Autodesk Inventor part; units mm, degrees
(part 2 of 3)
  line L383 (87.0601, -26.6576) -> (86.7601, -26.6576)
  line L384 (84.5601, -24.0434) -> (84.5601, -7.2718)
  line L385 (89.5601, -7.2718) -> (89.5601, -24.0434)
  arc A154 (84.853, -6.5647) -> (84.5601, -7.2718) centre (85.5601, -7.2718) ccw
  line L386 (84.853, -6.5647) -> (86.7601, -4.6576)
  line L387 (87.0601, -4.6576) -> (86.7601, -4.6576)
  line L388 (87.0601, -4.6576) -> (87.3601, -4.6576)
  arc A155 (89.5601, -7.2718) -> (89.2672, -6.5647) centre (88.5601, -7.2718) ccw
  line L389 (89.2672, -6.5647) -> (87.3601, -4.6576)
  arc A156 (114.0672, 0.0495) -> (114.3601, 0.7566) centre (113.3601, 0.7566) ccw
  arc A157 (109.3601, 0.7566) -> (109.653, 0.0495) centre (110.3601, 0.7566) ccw
  line L390 (114.0672, 0.0495) -> (112.1601, -1.8576)
  line L391 (109.653, 0.0495) -> (111.5601, -1.8576)
  line L392 (111.8601, -1.8576) -> (112.1601, -1.8576)
  line L393 (111.8601, -1.8576) -> (111.5601, -1.8576)
  line L394 (109.3601, 0.7566) -> (109.3601, 17.5282)
  line L395 (114.3601, 17.5282) -> (114.3601, 0.7566)
  arc A158 (109.653, 18.2353) -> (109.3601, 17.5282) centre (110.3601, 17.5282) ccw
  line L396 (109.653, 18.2353) -> (111.5601, 20.1424)
  line L397 (111.8601, 20.1424) -> (111.5601, 20.1424)
  line L398 (111.8601, 20.1424) -> (112.1601, 20.1424)
  arc A159 (114.3601, 17.5282) -> (114.0672, 18.2353) centre (113.3601, 17.5282) ccw
  line L399 (114.0672, 18.2353) -> (112.1601, 20.1424)
  arc A160 (114.0672, -24.7505) -> (114.3601, -24.0434) centre (113.3601, -24.0434) ccw
  arc A161 (109.3601, -24.0434) -> (109.653, -24.7505) centre (110.3601, -24.0434) ccw
  line L400 (114.0672, -24.7505) -> (112.1601, -26.6576)
  line L401 (109.653, -24.7505) -> (111.5601, -26.6576)
  line L402 (111.8601, -26.6576) -> (112.1601, -26.6576)
  line L403 (111.8601, -26.6576) -> (111.5601, -26.6576)
  line L404 (109.3601, -24.0434) -> (109.3601, -7.2718)
  line L405 (114.3601, -7.2718) -> (114.3601, -24.0434)
  arc A162 (109.653, -6.5647) -> (109.3601, -7.2718) centre (110.3601, -7.2718) ccw
  line L406 (109.653, -6.5647) -> (111.5601, -4.6576)
  line L407 (111.8601, -4.6576) -> (111.5601, -4.6576)
  line L408 (111.8601, -4.6576) -> (112.1601, -4.6576)
  arc A163 (114.3601, -7.2718) -> (114.0672, -6.5647) centre (113.3601, -7.2718) ccw
  line L409 (114.0672, -6.5647) -> (112.1601, -4.6576)
  arc A164 (90.3672, -30.2647) -> (91.0743, -30.5576) centre (91.0743, -29.5576) ccw
  arc A165 (91.0743, -25.5576) -> (90.3672, -25.8505) centre (91.0743, -26.5576) ccw
  line L410 (90.3672, -30.2647) -> (88.4601, -28.3576)
  line L411 (90.3672, -25.8505) -> (88.4601, -27.7576)
  line L412 (88.4601, -28.0576) -> (88.4601, -28.3576)
  line L413 (88.4601, -28.0576) -> (88.4601, -27.7576)
  line L414 (91.0743, -25.5576) -> (107.8459, -25.5576)
  line L415 (107.8459, -30.5576) -> (91.0743, -30.5576)
  arc A166 (108.553, -25.8505) -> (107.8459, -25.5576) centre (107.8459, -26.5576) ccw
  line L416 (108.553, -25.8505) -> (110.4601, -27.7576)
  line L417 (110.4601, -28.0576) -> (110.4601, -27.7576)
  line L418 (110.4601, -28.0576) -> (110.4601, -28.3576)
  arc A167 (107.8459, -30.5576) -> (108.553, -30.2647) centre (107.8459, -29.5576) ccw
  line L419 (108.553, -30.2647) -> (110.4601, -28.3576)
  line L420 (-45.8399, 8.0424) -> (-44.8399, 8.0424)
  line L421 (-44.8399, 8.0424) -> (-42.8399, 6.0424)
  line L422 (-42.8399, 6.0424) -> (-42.8399, 5.0424)
  line L423 (-42.8399, 5.0424) -> (-44.8399, 3.0424)
  line L424 (-44.8399, 3.0424) -> (-45.8399, 3.0424)
  line L425 (-45.8399, 3.0424) -> (-47.8399, 5.0424)
  line L426 (-47.8399, 5.0424) -> (-47.8399, 6.0424)
  line L427 (-47.8399, 6.0424) -> (-45.8399, 8.0424)
  line L428 (-45.8399, -11.9576) -> (-44.8399, -11.9576)
  line L429 (-44.8399, -11.9576) -> (-42.8399, -13.9576)
  line L430 (-42.8399, -13.9576) -> (-42.8399, -14.9576)
  line L431 (-42.8399, -14.9576) -> (-44.8399, -16.9576)
  line L432 (-44.8399, -16.9576) -> (-45.8399, -16.9576)
  line L433 (-45.8399, -16.9576) -> (-47.8399, -14.9576)
  line L434 (-47.8399, -14.9576) -> (-47.8399, -13.9576)
  line L435 (-47.8399, -13.9576) -> (-45.8399, -11.9576)
  line L436 (38.2601, 8.0424) -> (39.2601, 8.0424)
  line L437 (39.2601, 8.0424) -> (41.2601, 6.0424)
  line L438 (41.2601, 6.0424) -> (41.2601, 5.0424)
  line L439 (41.2601, 5.0424) -> (39.2601, 3.0424)
  line L440 (39.2601, 3.0424) -> (38.2601, 3.0424)
  line L441 (38.2601, 3.0424) -> (36.2601, 5.0424)
  line L442 (36.2601, 5.0424) -> (36.2601, 6.0424)
  line L443 (36.2601, 6.0424) -> (38.2601, 8.0424)
  line L444 (38.2601, -11.9576) -> (39.2601, -11.9576)
  line L445 (39.2601, -11.9576) -> (41.2601, -13.9576)
  line L446 (41.2601, -13.9576) -> (41.2601, -14.9576)
  line L447 (41.2601, -14.9576) -> (39.2601, -16.9576)
  line L448 (39.2601, -16.9576) -> (38.2601, -16.9576)
  line L449 (38.2601, -16.9576) -> (36.2601, -14.9576)
  line L450 (36.2601, -14.9576) -> (36.2601, -13.9576)
  line L451 (36.2601, -13.9576) -> (38.2601, -11.9576)
  arc A168 (-143.5328, -5.6647) -> (-142.8257, -5.9576) centre (-142.8257, -4.9576) ccw
  arc A169 (-142.8257, -0.9576) -> (-143.5328, -1.2505) centre (-142.8257, -1.9576) ccw
  line L452 (-143.5328, -5.6647) -> (-145.4399, -3.7576)
  line L453 (-145.4399, -3.4576) -> (-145.4399, -3.1576)
  line L454 (-145.4399, -3.4576) -> (-145.4399, -3.7576)
  line L455 (-143.5328, -1.2505) -> (-145.4399, -3.1576)
  line L456 (-142.8257, -0.9576) -> (-132.0541, -0.9576)
  line L457 (-132.0541, -5.9576) -> (-142.8257, -5.9576)
  arc A170 (-131.347, -1.2505) -> (-132.0541, -0.9576) centre (-132.0541, -1.9576) ccw
  arc A171 (-132.0541, -5.9576) -> (-131.347, -5.6647) centre (-132.0541, -4.9576) ccw
  line L458 (-131.347, -5.6647) -> (-129.4399, -3.7576)
  line L459 (-129.4399, -3.4576) -> (-129.4399, -3.7576)
  line L460 (-129.4399, -3.4576) -> (-129.4399, -3.1576)
  line L461 (-131.347, -1.2505) -> (-129.4399, -3.1576)
  arc A172 (-144.2328, -0.5505) -> (-143.9399, 0.1566) centre (-144.9399, 0.1566) ccw
  arc A173 (-148.9399, 0.1566) -> (-148.647, -0.5505) centre (-147.9399, 0.1566) ccw
  line L462 (-144.2328, -0.5505) -> (-146.1399, -2.4576)
  line L463 (-146.4399, -2.4576) -> (-146.7399, -2.4576)
  line L464 (-146.4399, -2.4576) -> (-146.1399, -2.4576)
  line L465 (-148.647, -0.5505) -> (-146.7399, -2.4576)
  line L466 (-148.9399, 0.1566) -> (-148.9399, 10.9282)
  line L467 (-143.9399, 10.9282) -> (-143.9399, 0.1566)
  arc A174 (-148.647, 11.6353) -> (-148.9399, 10.9282) centre (-147.9399, 10.9282) ccw
  arc A175 (-143.9399, 10.9282) -> (-144.2328, 11.6353) centre (-144.9399, 10.9282) ccw
  line L468 (-144.2328, 11.6353) -> (-146.1399, 13.5424)
  line L469 (-146.4399, 13.5424) -> (-146.1399, 13.5424)
  line L470 (-146.4399, 13.5424) -> (-146.7399, 13.5424)
  line L471 (-148.647, 11.6353) -> (-146.7399, 13.5424)
  arc A176 (-161.5328, -5.6647) -> (-160.8257, -5.9576) centre (-160.8257, -4.9576) ccw
  arc A177 (-160.8257, -0.9576) -> (-161.5328, -1.2505) centre (-160.8257, -1.9576) ccw
  line L472 (-161.5328, -5.6647) -> (-163.4399, -3.7576)
  line L473 (-163.4399, -3.4576) -> (-163.4399, -3.1576)
  line L474 (-163.4399, -3.4576) -> (-163.4399, -3.7576)
  line L475 (-161.5328, -1.2505) -> (-163.4399, -3.1576)
  line L476 (-160.8257, -0.9576) -> (-150.0541, -0.9576)
  line L477 (-150.0541, -5.9576) -> (-160.8257, -5.9576)
  arc A178 (-149.347, -1.2505) -> (-150.0541, -0.9576) centre (-150.0541, -1.9576) ccw
  arc A179 (-150.0541, -5.9576) -> (-149.347, -5.6647) centre (-150.0541, -4.9576) ccw
  line L478 (-149.347, -5.6647) -> (-147.4399, -3.7576)
  line L479 (-147.4399, -3.4576) -> (-147.4399, -3.7576)
  line L480 (-147.4399, -3.4576) -> (-147.4399, -3.1576)
  line L481 (-149.347, -1.2505) -> (-147.4399, -3.1576)
  arc A180 (-144.2328, -18.5505) -> (-143.9399, -17.8434) centre (-144.9399, -17.8434) ccw
  arc A181 (-148.9399, -17.8434) -> (-148.647, -18.5505) centre (-147.9399, -17.8434) ccw
  line L482 (-144.2328, -18.5505) -> (-146.1399, -20.4576)
  line L483 (-146.4399, -20.4576) -> (-146.7399, -20.4576)
  line L484 (-146.4399, -20.4576) -> (-146.1399, -20.4576)
  line L485 (-148.647, -18.5505) -> (-146.7399, -20.4576)
  line L486 (-148.9399, -17.8434) -> (-148.9399, -7.0718)
  line L487 (-143.9399, -7.0718) -> (-143.9399, -17.8434)
  arc A182 (-148.647, -6.3647) -> (-148.9399, -7.0718) centre (-147.9399, -7.0718) ccw
  arc A183 (-143.9399, -7.0718) -> (-144.2328, -6.3647) centre (-144.9399, -7.0718) ccw
  line L488 (-144.2328, -6.3647) -> (-146.1399, -4.4576)
  line L489 (-146.4399, -4.4576) -> (-146.1399, -4.4576)
  line L490 (-146.4399, -4.4576) -> (-146.7399, -4.4576)
  line L491 (-148.647, -6.3647) -> (-146.7399, -4.4576)
  arc A184 (-170.0328, 10.3353) -> (-169.3257, 10.0424) centre (-169.3257, 11.0424) ccw
  arc A185 (-169.3257, 15.0424) -> (-170.0328, 14.7495) centre (-169.3257, 14.0424) ccw
  line L492 (-170.0328, 10.3353) -> (-171.9399, 12.2424)
  line L493 (-171.9399, 12.5424) -> (-171.9399, 12.8424)
  line L494 (-171.9399, 12.5424) -> (-171.9399, 12.2424)
  line L495 (-170.0328, 14.7495) -> (-171.9399, 12.8424)
  line L496 (-169.3257, 15.0424) -> (-158.5541, 15.0424)
  line L497 (-158.5541, 10.0424) -> (-169.3257, 10.0424)
  arc A186 (-157.847, 14.7495) -> (-158.5541, 15.0424) centre (-158.5541, 14.0424) ccw
  arc A187 (-158.5541, 10.0424) -> (-157.847, 10.3353) centre (-158.5541, 11.0424) ccw
  line L498 (-157.847, 10.3353) -> (-155.9399, 12.2424)
  line L499 (-155.9399, 12.5424) -> (-155.9399, 12.2424)
  line L500 (-155.9399, 12.5424) -> (-155.9399, 12.8424)
  line L501 (-157.847, 14.7495) -> (-155.9399, 12.8424)
  arc A188 (-187.0328, 10.3353) -> (-186.3257, 10.0424) centre (-186.3257, 11.0424) ccw
  arc A189 (-186.3257, 15.0424) -> (-187.0328, 14.7495) centre (-186.3257, 14.0424) ccw
  line L502 (-187.0328, 10.3353) -> (-188.9399, 12.2424)
  line L503 (-188.9399, 12.5424) -> (-188.9399, 12.8424)
  line L504 (-188.9399, 12.5424) -> (-188.9399, 12.2424)
  line L505 (-187.0328, 14.7495) -> (-188.9399, 12.8424)
  line L506 (-186.3257, 15.0424) -> (-175.5541, 15.0424)
  line L507 (-175.5541, 10.0424) -> (-186.3257, 10.0424)
  arc A190 (-174.847, 14.7495) -> (-175.5541, 15.0424) centre (-175.5541, 14.0424) ccw
  arc A191 (-175.5541, 10.0424) -> (-174.847, 10.3353) centre (-175.5541, 11.0424) ccw
  line L508 (-174.847, 10.3353) -> (-172.9399, 12.2424)
  line L509 (-172.9399, 12.5424) -> (-172.9399, 12.2424)
  line L510 (-172.9399, 12.5424) -> (-172.9399, 12.8424)
  line L511 (-174.847, 14.7495) -> (-172.9399, 12.8424)
  arc A192 (-170.2328, -3.0647) -> (-169.9399, -2.3576) centre (-170.9399, -2.3576) ccw
  arc A193 (-174.9399, -2.3576) -> (-174.647, -3.0647) centre (-173.9399, -2.3576) ccw
  line L512 (-170.2328, -3.0647) -> (-172.1399, -4.9718)
  line L513 (-172.4399, -4.9718) -> (-172.7399, -4.9718)
  line L514 (-172.4399, -4.9718) -> (-172.1399, -4.9718)
  line L515 (-174.647, -3.0647) -> (-172.7399, -4.9718)
  line L516 (-174.9399, -2.3576) -> (-174.9399, 8.414)
  line L517 (-169.9399, 8.414) -> (-169.9399, -2.3576)
  arc A194 (-174.647, 9.1211) -> (-174.9399, 8.414) centre (-173.9399, 8.414) ccw
  arc A195 (-169.9399, 8.414) -> (-170.2328, 9.1211) centre (-170.9399, 8.414) ccw
  line L518 (-170.2328, 9.1211) -> (-172.1399, 11.0282)
  line L519 (-172.4399, 11.0282) -> (-172.1399, 11.0282)
  line L520 (-172.4399, 11.0282) -> (-172.7399, 11.0282)
  line L521 (-174.647, 9.1211) -> (-172.7399, 11.0282)
  arc A196 (-170.2328, -19.5647) -> (-169.9399, -18.8576) centre (-170.9399, -18.8576) ccw
  arc A197 (-174.9399, -18.8576) -> (-174.647, -19.5647) centre (-173.9399, -18.8576) ccw
  line L522 (-170.2328, -19.5647) -> (-172.1399, -21.4718)
  line L523 (-172.4399, -21.4718) -> (-172.7399, -21.4718)
  line L524 (-172.4399, -21.4718) -> (-172.1399, -21.4718)
  line L525 (-174.647, -19.5647) -> (-172.7399, -21.4718)
  line L526 (-174.9399, -18.8576) -> (-174.9399, -8.086)
  line L527 (-169.9399, -8.086) -> (-169.9399, -18.8576)
  arc A198 (-174.647, -7.3789) -> (-174.9399, -8.086) centre (-173.9399, -8.086) ccw
  arc A199 (-169.9399, -8.086) -> (-170.2328, -7.3789) centre (-170.9399, -8.086) ccw
  line L528 (-170.2328, -7.3789) -> (-172.1399, -5.4718)
  line L529 (-172.4399, -5.4718) -> (-172.1399, -5.4718)
  line L530 (-172.4399, -5.4718) -> (-172.7399, -5.4718)
  line L531 (-174.647, -7.3789) -> (-172.7399, -5.4718)
  point P0 (-22.4267, -1.12)
  dimension "d362" = 7.5
  dimension "d363" = 17
  dimension "d364" = 7.5
  dimension "d365" = 17
  dimension "d366" = 7.5
  dimension "d367" = 0
  dimension "d368" = 0
  dimension "d369" = 0
  dimension "d370" = 0
  dimension "d371" = 0
  dimension "d372" = 15
  dimension "d373" = 0
  dimension "d374" = 16
  dimension "d375" = 6
  dimension "d376" = 6
  dimension "d377" = 13.6
  dimension "d378" = 16
  dimension "d379" = 6
  dimension "d380" = 15
  dimension "d381" = 0
  dimension "d509" = 23
  dimension "d510" = 25
  dimension "d511" = 24.6
  dimension "d514" = 0.5
sketch "Clock Front Face Outline" plane through (0, 0, 0) normal (0, 0, 1) x (1, 0, 0)
  line L0 (-365.1075, -11.3808) -> (-85.1075, -11.3808)
  line L1 (-60.1075, -36.3808) -> (-60.1075, -56.3808)
  line L2 (-85.1075, -81.3808) -> (-365.1075, -81.3808)
  line L3 (-390.1075, -56.3808) -> (-390.1075, -36.3808)
  arc A0 (-365.1075, -11.3808) -> (-390.1075, -36.3808) centre (-365.1075, -36.3808) ccw
  arc A1 (-60.1075, -36.3808) -> (-85.1075, -11.3808) centre (-85.1075, -36.3808) ccw
  arc A2 (-85.1075, -81.3808) -> (-60.1075, -56.3808) centre (-85.1075, -56.3808) ccw
  arc A3 (-390.1075, -56.3808) -> (-365.1075, -81.3808) centre (-365.1075, -56.3808) ccw
  point P0 (0, -2.2581)
  dimension "d429" = 330
  dimension "d430" = 70
  dimension "d431" = 25
  measures "d429" distance between parallel lines of L1 L3
  measures "d430" distance between parallel lines of L2 L0
  measures "d431" radius of A0
sketch "Small Segmemt" plane through (0, 0, 0) normal (0, 0, 1) x (1, 0, 0)
  arc A0 (-247.3536, -9.433) -> (-246.6465, -9.7259) centre (-246.6465, -8.7259) ccw
  arc A1 (-246.6465, -4.7259) -> (-247.3536, -5.0187) centre (-246.6465, -5.7259) ccw
  line L0 (-247.3536, -9.433) -> (-249.2607, -7.5259)
  line L1 (-249.2607, -7.2259) -> (-249.2607, -6.9259)
  line L2 (-249.2607, -7.2259) -> (-249.2607, -7.5259)
  line L3 (-247.3536, -5.0187) -> (-249.2607, -6.9259)
  line L4 (-246.6465, -4.7259) -> (-235.875, -4.7259)
  line L5 (-235.875, -9.7259) -> (-246.6465, -9.7259)
  arc A2 (-235.1679, -5.0187) -> (-235.875, -4.7259) centre (-235.875, -5.7259) ccw
  arc A3 (-235.875, -9.7259) -> (-235.1679, -9.433) centre (-235.875, -8.7259) ccw
  line L6 (-235.1679, -9.433) -> (-233.2607, -7.5259)
  line L7 (-233.2607, -7.2259) -> (-233.2607, -7.5259)
  line L8 (-233.2607, -7.2259) -> (-233.2607, -6.9259)
  line L9 (-235.1679, -5.0187) -> (-233.2607, -6.9259)
  point P0 (-225.4266, -6.7349)
  point P1 (-247.0607, -4.7259)
  point P2 (-247.0607, -9.7259)
  point P3 (-235.4607, -4.7259)
  point P4 (-235.4607, -9.7259)
  dimension "d462" = 2.2
  dimension "d463" = 2.2
  dimension "d464" = 2.2
  dimension "d465" = 2.2
  dimension "d466" = 2.2
  dimension "d467" = 2.2
  dimension "d468" = 2.2
  dimension "d469" = 1
  dimension "d470" = 5
  dimension "d471" = 2.2
  dimension "d472" = 2.2
  dimension "d473" = 135
  dimension "d474" = 16
  dimension "d475" = 135
  dimension "d476" = 2.5
  dimension "d477" = 5
  dimension "d478" = 16
  dimension "d479" = 2.2
  dimension "d480" = 0.3
  dimension "d481" = 0.3
  dimension "d482" = 0.3
  dimension "d483" = 0.3
  measures "d462" horizontal distance of point (-247.061, -9.726) L0.end
  measures "d463" horizontal distance of L8.end point (-235.461, -4.726)
  measures "d464" horizontal distance of point (-247.061, -4.726) L1.end
  measures "d465" horizontal distance of L6.end point (-235.461, -9.726)
  measures "d466" horizontal distance of L6.end point (-235.461, -9.726)
  measures "d467" horizontal distance of point (-247.061, -4.726) L1.end
  measures "d468" horizontal distance of point (-247.061, -9.726) L0.end
  measures "d469" radius of A1
  measures "d470" distance of point (-235.461, -9.726) point (-235.461, -4.726)
  measures "d471" horizontal distance of L8.end point (-235.461, -4.726)
  measures "d472" horizontal distance of point (-235.461, -9.726) L7.start
  measures "d473" angle of L5 L6
  measures "d474" horizontal distance of L6.end L1.start
  measures "d475" angle of L4 L9
  measures "d476" vertical distance of L7.start point (-235.461, -9.726)
  measures "d477" distance between parallel lines of L5 L4
  measures "d478" distance of L1.start L7.start
  measures "d479" horizontal distance of point (-247.061, -4.726) L1.start
  measures "d480" distance of L7.start L8.end
  measures "d481" distance of L6.end L7.start
  measures "d482" distance of L1.end L1.start
  measures "d483" distance of L0.end L1.start
sketch "Sketch1" plane through (0, 0, 0) normal (0, 0, 1) x (1, 0, 0)
  line L0 (-365.1075, -11.3808) -> (-85.1075, -11.3808)
  line L1 (-60.1075, -36.3808) -> (-60.1075, -56.3808)
  line L2 (-85.1075, -81.3808) -> (-365.1075, -81.3808)
  line L3 (-390.1075, -56.3808) -> (-390.1075, -36.3808)
  arc A0 (-365.1075, -11.3808) -> (-390.1075, -36.3808) centre (-365.1075, -36.3808) ccw
  arc A1 (-60.1075, -36.3808) -> (-85.1075, -11.3808) centre (-85.1075, -36.3808) ccw
  arc A2 (-85.1075, -81.3808) -> (-60.1075, -56.3808) centre (-85.1075, -56.3808) ccw
  arc A3 (-390.1075, -56.3808) -> (-365.1075, -81.3808) centre (-365.1075, -56.3808) ccw
  point P0 (0, 0)
extrude "Extrusion1" add sketch "Sketch1" along normal blind 3
sketch "Sketch5" plane through (0, 0, 3) normal (0, 0, 1) x (1, 0, 0)
  line L0 (-85.1075, -11.3808) -> (-365.1075, -11.3808) projected
  line L1 (-365.1075, -81.3808) -> (-85.1075, -81.3808) projected
  line L2 (-390.1075, -36.3808) -> (-390.1075, -56.3808) projected
  line L3 (-60.1075, -56.3808) -> (-60.1075, -36.3808) projected
  arc A0 (-136.1004, -24.0879) -> (-135.3933, -24.3808) centre (-135.3933, -23.3808) ccw
  arc A1 (-135.3933, -19.3808) -> (-136.1004, -19.6736) centre (-135.3933, -20.3808) ccw
  line L4 (-136.1004, -24.0879) -> (-138.0075, -22.1808)
  line L5 (-136.1004, -19.6736) -> (-138.0075, -21.5808)
  line L6 (-138.0075, -21.8808) -> (-138.0075, -22.1808)
  line L7 (-138.0075, -21.8808) -> (-138.0075, -21.5808)
  line L8 (-135.3933, -19.3808) -> (-118.6217, -19.3808)
  line L9 (-118.6217, -24.3808) -> (-135.3933, -24.3808)
  arc A2 (-117.9146, -19.6736) -> (-118.6217, -19.3808) centre (-118.6217, -20.3808) ccw
  line L10 (-117.9146, -19.6736) -> (-116.0075, -21.5808)
  line L11 (-116.0075, -21.8808) -> (-116.0075, -21.5808)
  line L12 (-116.0075, -21.8808) -> (-116.0075, -22.1808)
  arc A3 (-118.6217, -24.3808) -> (-117.9146, -24.0879) centre (-118.6217, -23.3808) ccw
  line L13 (-117.9146, -24.0879) -> (-116.0075, -22.1808)
  arc A4 (-136.1004, -48.8879) -> (-135.3933, -49.1808) centre (-135.3933, -48.1808) ccw
  arc A5 (-135.3933, -44.1808) -> (-136.1004, -44.4736) centre (-135.3933, -45.1808) ccw
  line L14 (-136.1004, -48.8879) -> (-138.0075, -46.9808)
  line L15 (-136.1004, -44.4736) -> (-138.0075, -46.3808)
  line L16 (-138.0075, -46.6808) -> (-138.0075, -46.9808)
  line L17 (-138.0075, -46.6808) -> (-138.0075, -46.3808)
  line L18 (-135.3933, -44.1808) -> (-118.6217, -44.1808)
  line L19 (-118.6217, -49.1808) -> (-135.3933, -49.1808)
  arc A6 (-117.9146, -44.4736) -> (-118.6217, -44.1808) centre (-118.6217, -45.1808) ccw
  line L20 (-117.9146, -44.4736) -> (-116.0075, -46.3808)
  line L21 (-116.0075, -46.6808) -> (-116.0075, -46.3808)
  line L22 (-116.0075, -46.6808) -> (-116.0075, -46.9808)
  arc A7 (-118.6217, -49.1808) -> (-117.9146, -48.8879) centre (-118.6217, -48.1808) ccw
  line L23 (-117.9146, -48.8879) -> (-116.0075, -46.9808)
  arc A8 (-137.2004, -43.3736) -> (-136.9075, -42.6665) centre (-137.9075, -42.6665) ccw
  arc A9 (-141.9075, -42.6665) -> (-141.6146, -43.3736) centre (-140.9075, -42.6665) ccw
  line L24 (-137.2004, -43.3736) -> (-139.1075, -45.2808)
  line L25 (-141.6146, -43.3736) -> (-139.7075, -45.2808)
  line L26 (-139.4075, -45.2808) -> (-139.1075, -45.2808)
  line L27 (-139.4075, -45.2808) -> (-139.7075, -45.2808)
  line L28 (-141.9075, -42.6665) -> (-141.9075, -25.895)
  line L29 (-136.9075, -25.895) -> (-136.9075, -42.6665)
  arc A10 (-141.6146, -25.1879) -> (-141.9075, -25.895) centre (-140.9075, -25.895) ccw
  line L30 (-141.6146, -25.1879) -> (-139.7075, -23.2808)
  line L31 (-139.4075, -23.2808) -> (-139.7075, -23.2808)
  line L32 (-139.4075, -23.2808) -> (-139.1075, -23.2808)
  arc A11 (-136.9075, -25.895) -> (-137.2004, -25.1879) centre (-137.9075, -25.895) ccw
  line L33 (-137.2004, -25.1879) -> (-139.1075, -23.2808)
  arc A12 (-137.2004, -68.1736) -> (-136.9075, -67.4665) centre (-137.9075, -67.4665) ccw
  arc A13 (-141.9075, -67.4665) -> (-141.6146, -68.1736) centre (-140.9075, -67.4665) ccw
  line L34 (-137.2004, -68.1736) -> (-139.1075, -70.0808)
  line L35 (-141.6146, -68.1736) -> (-139.7075, -70.0808)
  line L36 (-139.4075, -70.0808) -> (-139.1075, -70.0808)
  line L37 (-139.4075, -70.0808) -> (-139.7075, -70.0808)
  line L38 (-141.9075, -67.4665) -> (-141.9075, -50.695)
  line L39 (-136.9075, -50.695) -> (-136.9075, -67.4665)
  arc A14 (-141.6146, -49.9879) -> (-141.9075, -50.695) centre (-140.9075, -50.695) ccw
  line L40 (-141.6146, -49.9879) -> (-139.7075, -48.0808)
  line L41 (-139.4075, -48.0808) -> (-139.7075, -48.0808)
  line L42 (-139.4075, -48.0808) -> (-139.1075, -48.0808)
  arc A15 (-136.9075, -50.695) -> (-137.2004, -49.9879) centre (-137.9075, -50.695) ccw
  line L43 (-137.2004, -49.9879) -> (-139.1075, -48.0808)
  arc A16 (-112.4004, -43.3736) -> (-112.1075, -42.6665) centre (-113.1075, -42.6665) ccw
  arc A17 (-117.1075, -42.6665) -> (-116.8146, -43.3736) centre (-116.1075, -42.6665) ccw
  line L44 (-112.4004, -43.3736) -> (-114.3075, -45.2808)
  line L45 (-116.8146, -43.3736) -> (-114.9075, -45.2808)
  line L46 (-114.6075, -45.2808) -> (-114.3075, -45.2808)
  line L47 (-114.6075, -45.2808) -> (-114.9075, -45.2808)
  line L48 (-117.1075, -42.6665) -> (-117.1075, -25.895)
  line L49 (-112.1075, -25.895) -> (-112.1075, -42.6665)
  arc A18 (-116.8146, -25.1879) -> (-117.1075, -25.895) centre (-116.1075, -25.895) ccw
  line L50 (-116.8146, -25.1879) -> (-114.9075, -23.2808)
  line L51 (-114.6075, -23.2808) -> (-114.9075, -23.2808)
  line L52 (-114.6075, -23.2808) -> (-114.3075, -23.2808)
  arc A19 (-112.1075, -25.895) -> (-112.4004, -25.1879) centre (-113.1075, -25.895) ccw
  line L53 (-112.4004, -25.1879) -> (-114.3075, -23.2808)
  arc A20 (-112.4004, -68.1736) -> (-112.1075, -67.4665) centre (-113.1075, -67.4665) ccw
  arc A21 (-117.1075, -67.4665) -> (-116.8146, -68.1736) centre (-116.1075, -67.4665) ccw
  line L54 (-112.4004, -68.1736) -> (-114.3075, -70.0808)
  line L55 (-116.8146, -68.1736) -> (-114.9075, -70.0808)
  line L56 (-114.6075, -70.0808) -> (-114.3075, -70.0808)
  line L57 (-114.6075, -70.0808) -> (-114.9075, -70.0808)
  line L58 (-117.1075, -67.4665) -> (-117.1075, -50.695)
  line L59 (-112.1075, -50.695) -> (-112.1075, -67.4665)
  arc A22 (-116.8146, -49.9879) -> (-117.1075, -50.695) centre (-116.1075, -50.695) ccw
  line L60 (-116.8146, -49.9879) -> (-114.9075, -48.0808)
  line L61 (-114.6075, -48.0808) -> (-114.9075, -48.0808)
  line L62 (-114.6075, -48.0808) -> (-114.3075, -48.0808)
  arc A23 (-112.1075, -50.695) -> (-112.4004, -49.9879) centre (-113.1075, -50.695) ccw
  line L63 (-112.4004, -49.9879) -> (-114.3075, -48.0808)
  arc A24 (-136.1004, -73.6879) -> (-135.3933, -73.9808) centre (-135.3933, -72.9808) ccw
  arc A25 (-135.3933, -68.9808) -> (-136.1004, -69.2736) centre (-135.3933, -69.9808) ccw
  line L64 (-136.1004, -73.6879) -> (-138.0075, -71.7808)
  line L65 (-136.1004, -69.2736) -> (-138.0075, -71.1808)
  line L66 (-138.0075, -71.4808) -> (-138.0075, -71.7808)
  line L67 (-138.0075, -71.4808) -> (-138.0075, -71.1808)
  line L68 (-135.3933, -68.9808) -> (-118.6217, -68.9808)
  line L69 (-118.6217, -73.9808) -> (-135.3933, -73.9808)
  arc A26 (-117.9146, -69.2736) -> (-118.6217, -68.9808) centre (-118.6217, -69.9808) ccw
  line L70 (-117.9146, -69.2736) -> (-116.0075, -71.1808)
  line L71 (-116.0075, -71.4808) -> (-116.0075, -71.1808)
  line L72 (-116.0075, -71.4808) -> (-116.0075, -71.7808)
  arc A27 (-118.6217, -73.9808) -> (-117.9146, -73.6879) centre (-118.6217, -72.9808) ccw
  line L73 (-117.9146, -73.6879) -> (-116.0075, -71.7808)
  arc A28 (-182.9004, -24.0879) -> (-182.1933, -24.3808) centre (-182.1933, -23.3808) ccw
  arc A29 (-182.1933, -19.3808) -> (-182.9004, -19.6736) centre (-182.1933, -20.3808) ccw
  line L74 (-182.9004, -24.0879) -> (-184.8075, -22.1808)
  line L75 (-182.9004, -19.6736) -> (-184.8075, -21.5808)
  line L76 (-184.8075, -21.8808) -> (-184.8075, -22.1808)
  line L77 (-184.8075, -21.8808) -> (-184.8075, -21.5808)
  line L78 (-182.1933, -19.3808) -> (-165.4217, -19.3808)
  line L79 (-165.4217, -24.3808) -> (-182.1933, -24.3808)
  arc A30 (-164.7146, -19.6736) -> (-165.4217, -19.3808) centre (-165.4217, -20.3808) ccw
  line L80 (-164.7146, -19.6736) -> (-162.8075, -21.5808)
  line L81 (-162.8075, -21.8808) -> (-162.8075, -21.5808)
  line L82 (-162.8075, -21.8808) -> (-162.8075, -22.1808)
  arc A31 (-165.4217, -24.3808) -> (-164.7146, -24.0879) centre (-165.4217, -23.3808) ccw
  line L83 (-164.7146, -24.0879) -> (-162.8075, -22.1808)
  arc A32 (-182.9004, -48.8879) -> (-182.1933, -49.1808) centre (-182.1933, -48.1808) ccw
  arc A33 (-182.1933, -44.1808) -> (-182.9004, -44.4736) centre (-182.1933, -45.1808) ccw
  line L84 (-182.9004, -48.8879) -> (-184.8075, -46.9808)
  line L85 (-182.9004, -44.4736) -> (-184.8075, -46.3808)
  line L86 (-184.8075, -46.6808) -> (-184.8075, -46.9808)
  line L87 (-184.8075, -46.6808) -> (-184.8075, -46.3808)
  line L88 (-182.1933, -44.1808) -> (-165.4217, -44.1808)
  line L89 (-165.4217, -49.1808) -> (-182.1933, -49.1808)
  arc A34 (-164.7146, -44.4736) -> (-165.4217, -44.1808) centre (-165.4217, -45.1808) ccw
  line L90 (-164.7146, -44.4736) -> (-162.8075, -46.3808)
  line L91 (-162.8075, -46.6808) -> (-162.8075, -46.3808)
  line L92 (-162.8075, -46.6808) -> (-162.8075, -46.9808)
  arc A35 (-165.4217, -49.1808) -> (-164.7146, -48.8879) centre (-165.4217, -48.1808) ccw
  line L93 (-164.7146, -48.8879) -> (-162.8075, -46.9808)
  arc A36 (-184.0004, -43.3736) -> (-183.7075, -42.6665) centre (-184.7075, -42.6665) ccw
  arc A37 (-188.7075, -42.6665) -> (-188.4146, -43.3736) centre (-187.7075, -42.6665) ccw
  line L94 (-184.0004, -43.3736) -> (-185.9075, -45.2808)
  line L95 (-188.4146, -43.3736) -> (-186.5075, -45.2808)
  line L96 (-186.2075, -45.2808) -> (-185.9075, -45.2808)
  line L97 (-186.2075, -45.2808) -> (-186.5075, -45.2808)
  line L98 (-188.7075, -42.6665) -> (-188.7075, -25.895)
  line L99 (-183.7075, -25.895) -> (-183.7075, -42.6665)
  arc A38 (-188.4146, -25.1879) -> (-188.7075, -25.895) centre (-187.7075, -25.895) ccw
  line L100 (-188.4146, -25.1879) -> (-186.5075, -23.2808)
  line L101 (-186.2075, -23.2808) -> (-186.5075, -23.2808)
  line L102 (-186.2075, -23.2808) -> (-185.9075, -23.2808)
  arc A39 (-183.7075, -25.895) -> (-184.0004, -25.1879) centre (-184.7075, -25.895) ccw
  line L103 (-184.0004, -25.1879) -> (-185.9075, -23.2808)
  arc A40 (-184.0004, -68.1736) -> (-183.7075, -67.4665) centre (-184.7075, -67.4665) ccw
  arc A41 (-188.7075, -67.4665) -> (-188.4146, -68.1736) centre (-187.7075, -67.4665) ccw
  line L104 (-184.0004, -68.1736) -> (-185.9075, -70.0808)
  line L105 (-188.4146, -68.1736) -> (-186.5075, -70.0808)
  line L106 (-186.2075, -70.0808) -> (-185.9075, -70.0808)
  line L107 (-186.2075, -70.0808) -> (-186.5075, -70.0808)
  line L108 (-188.7075, -67.4665) -> (-188.7075, -50.695)
  line L109 (-183.7075, -50.695) -> (-183.7075, -67.4665)
  arc A42 (-188.4146, -49.9879) -> (-188.7075, -50.695) centre (-187.7075, -50.695) ccw
  line L110 (-188.4146, -49.9879) -> (-186.5075, -48.0808)
  line L111 (-186.2075, -48.0808) -> (-186.5075, -48.0808)
  line L112 (-186.2075, -48.0808) -> (-185.9075, -48.0808)
  arc A43 (-183.7075, -50.695) -> (-184.0004, -49.9879) centre (-184.7075, -50.695) ccw
  line L113 (-184.0004, -49.9879) -> (-185.9075, -48.0808)
  arc A44 (-159.2004, -43.3736) -> (-158.9075, -42.6665) centre (-159.9075, -42.6665) ccw
  arc A45 (-163.9075, -42.6665) -> (-163.6146, -43.3736) centre (-162.9075, -42.6665) ccw
  line L114 (-159.2004, -43.3736) -> (-161.1075, -45.2808)
  line L115 (-163.6146, -43.3736) -> (-161.7075, -45.2808)
  line L116 (-161.4075, -45.2808) -> (-161.1075, -45.2808)
  line L117 (-161.4075, -45.2808) -> (-161.7075, -45.2808)
  line L118 (-163.9075, -42.6665) -> (-163.9075, -25.895)
  line L119 (-158.9075, -25.895) -> (-158.9075, -42.6665)
  arc A46 (-163.6146, -25.1879) -> (-163.9075, -25.895) centre (-162.9075, -25.895) ccw
  line L120 (-163.6146, -25.1879) -> (-161.7075, -23.2808)
  line L121 (-161.4075, -23.2808) -> (-161.7075, -23.2808)
  line L122 (-161.4075, -23.2808) -> (-161.1075, -23.2808)
  arc A47 (-158.9075, -25.895) -> (-159.2004, -25.1879) centre (-159.9075, -25.895) ccw
  line L123 (-159.2004, -25.1879) -> (-161.1075, -23.2808)
  arc A48 (-159.2004, -68.1736) -> (-158.9075, -67.4665) centre (-159.9075, -67.4665) ccw
  arc A49 (-163.9075, -67.4665) -> (-163.6146, -68.1736) centre (-162.9075, -67.4665) ccw
  line L124 (-159.2004, -68.1736) -> (-161.1075, -70.0808)
  line L125 (-163.6146, -68.1736) -> (-161.7075, -70.0808)
  line L126 (-161.4075, -70.0808) -> (-161.1075, -70.0808)
  line L127 (-161.4075, -70.0808) -> (-161.7075, -70.0808)
  line L128 (-163.9075, -67.4665) -> (-163.9075, -50.695)
  line L129 (-158.9075, -50.695) -> (-158.9075, -67.4665)
  arc A50 (-163.6146, -49.9879) -> (-163.9075, -50.695) centre (-162.9075, -50.695) ccw
  line L130 (-163.6146, -49.9879) -> (-161.7075, -48.0808)
  line L131 (-161.4075, -48.0808) -> (-161.7075, -48.0808)
  line L132 (-161.4075, -48.0808) -> (-161.1075, -48.0808)
  arc A51 (-158.9075, -50.695) -> (-159.2004, -49.9879) centre (-159.9075, -50.695) ccw
  line L133 (-159.2004, -49.9879) -> (-161.1075, -48.0808)
  arc A52 (-182.9004, -73.6879) -> (-182.1933, -73.9808) centre (-182.1933, -72.9808) ccw
  arc A53 (-182.1933, -68.9808) -> (-182.9004, -69.2736) centre (-182.1933, -69.9808) ccw
  line L134 (-182.9004, -73.6879) -> (-184.8075, -71.7808)
  line L135 (-182.9004, -69.2736) -> (-184.8075, -71.1808)
  line L136 (-184.8075, -71.4808) -> (-184.8075, -71.7808)
  line L137 (-184.8075, -71.4808) -> (-184.8075, -71.1808)
  line L138 (-182.1933, -68.9808) -> (-165.4217, -68.9808)
  line L139 (-165.4217, -73.9808) -> (-182.1933, -73.9808)
  arc A54 (-164.7146, -69.2736) -> (-165.4217, -68.9808) centre (-165.4217, -69.9808) ccw
  line L140 (-164.7146, -69.2736) -> (-162.8075, -71.1808)
  line L141 (-162.8075, -71.4808) -> (-162.8075, -71.1808)
  line L142 (-162.8075, -71.4808) -> (-162.8075, -71.7808)
  arc A55 (-165.4217, -73.9808) -> (-164.7146, -73.6879) centre (-165.4217, -72.9808) ccw
  line L143 (-164.7146, -73.6879) -> (-162.8075, -71.7808)
  arc A56 (-220.2004, -24.0879) -> (-219.4933, -24.3808) centre (-219.4933, -23.3808) ccw
  arc A57 (-219.4933, -19.3808) -> (-220.2004, -19.6736) centre (-219.4933, -20.3808) ccw
  line L144 (-220.2004, -24.0879) -> (-222.1075, -22.1808)
  line L145 (-220.2004, -19.6736) -> (-222.1075, -21.5808)
  line L146 (-222.1075, -21.8808) -> (-222.1075, -22.1808)
  line L147 (-222.1075, -21.8808) -> (-222.1075, -21.5808)
  line L148 (-219.4933, -19.3808) -> (-202.7217, -19.3808)
  line L149 (-202.7217, -24.3808) -> (-219.4933, -24.3808)
  arc A58 (-202.0146, -19.6736) -> (-202.7217, -19.3808) centre (-202.7217, -20.3808) ccw
  line L150 (-202.0146, -19.6736) -> (-200.1075, -21.5808)
  line L151 (-200.1075, -21.8808) -> (-200.1075, -21.5808)
  line L152 (-200.1075, -21.8808) -> (-200.1075, -22.1808)
  arc A59 (-202.7217, -24.3808) -> (-202.0146, -24.0879) centre (-202.7217, -23.3808) ccw
  line L153 (-202.0146, -24.0879) -> (-200.1075, -22.1808)
  arc A60 (-220.2004, -48.8879) -> (-219.4933, -49.1808) centre (-219.4933, -48.1808) ccw
  arc A61 (-219.4933, -44.1808) -> (-220.2004, -44.4736) centre (-219.4933, -45.1808) ccw
  line L154 (-220.2004, -48.8879) -> (-222.1075, -46.9808)
  line L155 (-220.2004, -44.4736) -> (-222.1075, -46.3808)
  line L156 (-222.1075, -46.6808) -> (-222.1075, -46.9808)
  line L157 (-222.1075, -46.6808) -> (-222.1075, -46.3808)
  line L158 (-219.4933, -44.1808) -> (-202.7217, -44.1808)
  line L159 (-202.7217, -49.1808) -> (-219.4933, -49.1808)
  arc A62 (-202.0146, -44.4736) -> (-202.7217, -44.1808) centre (-202.7217, -45.1808) ccw
  line L160 (-202.0146, -44.4736) -> (-200.1075, -46.3808)
  line L161 (-200.1075, -46.6808) -> (-200.1075, -46.3808)
  line L162 (-200.1075, -46.6808) -> (-200.1075, -46.9808)
  arc A63 (-202.7217, -49.1808) -> (-202.0146, -48.8879) centre (-202.7217, -48.1808) ccw
  line L163 (-202.0146, -48.8879) -> (-200.1075, -46.9808)
  arc A64 (-221.3004, -43.3736) -> (-221.0075, -42.6665) centre (-222.0075, -42.6665) ccw
  arc A65 (-226.0075, -42.6665) -> (-225.7146, -43.3736) centre (-225.0075, -42.6665) ccw
  line L164 (-221.3004, -43.3736) -> (-223.2075, -45.2808)
  line L165 (-225.7146, -43.3736) -> (-223.8075, -45.2808)
  line L166 (-223.5075, -45.2808) -> (-223.2075, -45.2808)
  line L167 (-223.5075, -45.2808) -> (-223.8075, -45.2808)
  line L168 (-226.0075, -42.6665) -> (-226.0075, -25.895)
  line L169 (-221.0075, -25.895) -> (-221.0075, -42.6665)
  arc A66 (-225.7146, -25.1879) -> (-226.0075, -25.895) centre (-225.0075, -25.895) ccw
  line L170 (-225.7146, -25.1879) -> (-223.8075, -23.2808)
  line L171 (-223.5075, -23.2808) -> (-223.8075, -23.2808)
  line L172 (-223.5075, -23.2808) -> (-223.2075, -23.2808)
  arc A67 (-221.0075, -25.895) -> (-221.3004, -25.1879) centre (-222.0075, -25.895) ccw
  line L173 (-221.3004, -25.1879) -> (-223.2075, -23.2808)
  arc A68 (-221.3004, -68.1736) -> (-221.0075, -67.4665) centre (-222.0075, -67.4665) ccw
  arc A69 (-226.0075, -67.4665) -> (-225.7146, -68.1736) centre (-225.0075, -67.4665) ccw
  line L174 (-221.3004, -68.1736) -> (-223.2075, -70.0808)
  line L175 (-225.7146, -68.1736) -> (-223.8075, -70.0808)
  line L176 (-223.5075, -70.0808) -> (-223.2075, -70.0808)
  line L177 (-223.5075, -70.0808) -> (-223.8075, -70.0808)
  line L178 (-226.0075, -67.4665) -> (-226.0075, -50.695)
  line L179 (-221.0075, -50.695) -> (-221.0075, -67.4665)
  arc A70 (-225.7146, -49.9879) -> (-226.0075, -50.695) centre (-225.0075, -50.695) ccw
  line L180 (-225.7146, -49.9879) -> (-223.8075, -48.0808)
  line L181 (-223.5075, -48.0808) -> (-223.8075, -48.0808)
  line L182 (-223.5075, -48.0808) -> (-223.2075, -48.0808)
  arc A71 (-221.0075, -50.695) -> (-221.3004, -49.9879) centre (-222.0075, -50.695) ccw
  line L183 (-221.3004, -49.9879) -> (-223.2075, -48.0808)
  arc A72 (-196.5004, -43.3736) -> (-196.2075, -42.6665) centre (-197.2075, -42.6665) ccw
  arc A73 (-201.2075, -42.6665) -> (-200.9146, -43.3736) centre (-200.2075, -42.6665) ccw
  line L184 (-196.5004, -43.3736) -> (-198.4075, -45.2808)
  line L185 (-200.9146, -43.3736) -> (-199.0075, -45.2808)
  line L186 (-198.7075, -45.2808) -> (-198.4075, -45.2808)
  line L187 (-198.7075, -45.2808) -> (-199.0075, -45.2808)
  line L188 (-201.2075, -42.6665) -> (-201.2075, -25.895)
  line L189 (-196.2075, -25.895) -> (-196.2075, -42.6665)
  arc A74 (-200.9146, -25.1879) -> (-201.2075, -25.895) centre (-200.2075, -25.895) ccw
  line L190 (-200.9146, -25.1879) -> (-199.0075, -23.2808)
  line L191 (-198.7075, -23.2808) -> (-199.0075, -23.2808)
  line L192 (-198.7075, -23.2808) -> (-198.4075, -23.2808)
  arc A75 (-196.2075, -25.895) -> (-196.5004, -25.1879) centre (-197.2075, -25.895) ccw
  line L193 (-196.5004, -25.1879) -> (-198.4075, -23.2808)
  arc A76 (-196.5004, -68.1736) -> (-196.2075, -67.4665) centre (-197.2075, -67.4665) ccw
  arc A77 (-201.2075, -67.4665) -> (-200.9146, -68.1736) centre (-200.2075, -67.4665) ccw
  line L194 (-196.5004, -68.1736) -> (-198.4075, -70.0808)
  line L195 (-200.9146, -68.1736) -> (-199.0075, -70.0808)
  line L196 (-198.7075, -70.0808) -> (-198.4075, -70.0808)
  line L197 (-198.7075, -70.0808) -> (-199.0075, -70.0808)
  line L198 (-201.2075, -67.4665) -> (-201.2075, -50.695)
  line L199 (-196.2075, -50.695) -> (-196.2075, -67.4665)
  arc A78 (-200.9146, -49.9879) -> (-201.2075, -50.695) centre (-200.2075, -50.695) ccw
  line L200 (-200.9146, -49.9879) -> (-199.0075, -48.0808)
  line L201 (-198.7075, -48.0808) -> (-199.0075, -48.0808)
  line L202 (-198.7075, -48.0808) -> (-198.4075, -48.0808)
  arc A79 (-196.2075, -50.695) -> (-196.5004, -49.9879) centre (-197.2075, -50.695) ccw
  line L203 (-196.5004, -49.9879) -> (-198.4075, -48.0808)
  arc A80 (-220.2004, -73.6879) -> (-219.4933, -73.9808) centre (-219.4933, -72.9808) ccw
  arc A81 (-219.4933, -68.9808) -> (-220.2004, -69.2736) centre (-219.4933, -69.9808) ccw
  line L204 (-220.2004, -73.6879) -> (-222.1075, -71.7808)
  line L205 (-220.2004, -69.2736) -> (-222.1075, -71.1808)
  line L206 (-222.1075, -71.4808) -> (-222.1075, -71.7808)
  line L207 (-222.1075, -71.4808) -> (-222.1075, -71.1808)
  line L208 (-219.4933, -68.9808) -> (-202.7217, -68.9808)
  line L209 (-202.7217, -73.9808) -> (-219.4933, -73.9808)
  arc A82 (-202.0146, -69.2736) -> (-202.7217, -68.9808) centre (-202.7217, -69.9808) ccw
  line L210 (-202.0146, -69.2736) -> (-200.1075, -71.1808)
  line L211 (-200.1075, -71.4808) -> (-200.1075, -71.1808)
  line L212 (-200.1075, -71.4808) -> (-200.1075, -71.7808)
  arc A83 (-202.7217, -73.9808) -> (-202.0146, -73.6879) centre (-202.7217, -72.9808) ccw
  line L213 (-202.0146, -73.6879) -> (-200.1075, -71.7808)
  arc A84 (-267.0004, -24.0879) -> (-266.2933, -24.3808) centre (-266.2933, -23.3808) ccw
  arc A85 (-266.2933, -19.3808) -> (-267.0004, -19.6736) centre (-266.2933, -20.3808) ccw
  line L214 (-267.0004, -24.0879) -> (-268.9075, -22.1808)
  line L215 (-267.0004, -19.6736) -> (-268.9075, -21.5808)
  line L216 (-268.9075, -21.8808) -> (-268.9075, -22.1808)
  line L217 (-268.9075, -21.8808) -> (-268.9075, -21.5808)
  line L218 (-266.2933, -19.3808) -> (-249.5217, -19.3808)
  line L219 (-249.5217, -24.3808) -> (-266.2933, -24.3808)
  arc A86 (-248.8146, -19.6736) -> (-249.5217, -19.3808) centre (-249.5217, -20.3808) ccw
  line L220 (-248.8146, -19.6736) -> (-246.9075, -21.5808)
  line L221 (-246.9075, -21.8808) -> (-246.9075, -21.5808)
  line L222 (-246.9075, -21.8808) -> (-246.9075, -22.1808)
  arc A87 (-249.5217, -24.3808) -> (-248.8146, -24.0879) centre (-249.5217, -23.3808) ccw
  line L223 (-248.8146, -24.0879) -> (-246.9075, -22.1808)
  arc A88 (-267.0004, -48.8879) -> (-266.2933, -49.1808) centre (-266.2933, -48.1808) ccw
  arc A89 (-266.2933, -44.1808) -> (-267.0004, -44.4736) centre (-266.2933, -45.1808) ccw
  line L224 (-267.0004, -48.8879) -> (-268.9075, -46.9808)
  line L225 (-267.0004, -44.4736) -> (-268.9075, -46.3808)
  line L226 (-268.9075, -46.6808) -> (-268.9075, -46.9808)
  line L227 (-268.9075, -46.6808) -> (-268.9075, -46.3808)
  line L228 (-266.2933, -44.1808) -> (-249.5217, -44.1808)
  line L229 (-249.5217, -49.1808) -> (-266.2933, -49.1808)
  arc A90 (-248.8146, -44.4736) -> (-249.5217, -44.1808) centre (-249.5217, -45.1808) ccw
  line L230 (-248.8146, -44.4736) -> (-246.9075, -46.3808)
  line L231 (-246.9075, -46.6808) -> (-246.9075, -46.3808)
  line L232 (-246.9075, -46.6808) -> (-246.9075, -46.9808)
  arc A91 (-249.5217, -49.1808) -> (-248.8146, -48.8879) centre (-249.5217, -48.1808) ccw
  line L233 (-248.8146, -48.8879) -> (-246.9075, -46.9808)
  arc A92 (-268.1004, -43.3736) -> (-267.8075, -42.6665) centre (-268.8075, -42.6665) ccw
  arc A93 (-272.8075, -42.6665) -> (-272.5146, -43.3736) centre (-271.8075, -42.6665) ccw
  line L234 (-268.1004, -43.3736) -> (-270.0075, -45.2808)
  line L235 (-272.5146, -43.3736) -> (-270.6075, -45.2808)
  line L236 (-270.3075, -45.2808) -> (-270.0075, -45.2808)
  line L237 (-270.3075, -45.2808) -> (-270.6075, -45.2808)
  line L238 (-272.8075, -42.6665) -> (-272.8075, -25.895)
  line L239 (-267.8075, -25.895) -> (-267.8075, -42.6665)
  arc A94 (-272.5146, -25.1879) -> (-272.8075, -25.895) centre (-271.8075, -25.895) ccw
  line L240 (-272.5146, -25.1879) -> (-270.6075, -23.2808)
  line L241 (-270.3075, -23.2808) -> (-270.6075, -23.2808)
  line L242 (-270.3075, -23.2808) -> (-270.0075, -23.2808)
  arc A95 (-267.8075, -25.895) -> (-268.1004, -25.1879) centre (-268.8075, -25.895) ccw
  line L243 (-268.1004, -25.1879) -> (-270.0075, -23.2808)
  arc A96 (-268.1004, -68.1736) -> (-267.8075, -67.4665) centre (-268.8075, -67.4665) ccw
  arc A97 (-272.8075, -67.4665) -> (-272.5146, -68.1736) centre (-271.8075, -67.4665) ccw
  line L244 (-268.1004, -68.1736) -> (-270.0075, -70.0808)
  line L245 (-272.5146, -68.1736) -> (-270.6075, -70.0808)
  line L246 (-270.3075, -70.0808) -> (-270.0075, -70.0808)
  line L247 (-270.3075, -70.0808) -> (-270.6075, -70.0808)
  line L248 (-272.8075, -67.4665) -> (-272.8075, -50.695)
  line L249 (-267.8075, -50.695) -> (-267.8075, -67.4665)
  arc A98 (-272.5146, -49.9879) -> (-272.8075, -50.695) centre (-271.8075, -50.695) ccw
  line L250 (-272.5146, -49.9879) -> (-270.6075, -48.0808)
  line L251 (-270.3075, -48.0808) -> (-270.6075, -48.0808)
  line L252 (-270.3075, -48.0808) -> (-270.0075, -48.0808)
  arc A99 (-267.8075, -50.695) -> (-268.1004, -49.9879) centre (-268.8075, -50.695) ccw
  line L253 (-268.1004, -49.9879) -> (-270.0075, -48.0808)
  arc A100 (-243.3004, -43.3736) -> (-243.0075, -42.6665) centre (-244.0075, -42.6665) ccw
  arc A101 (-248.0075, -42.6665) -> (-247.7146, -43.3736) centre (-247.0075, -42.6665) ccw
  line L254 (-243.3004, -43.3736) -> (-245.2075, -45.2808)
  line L255 (-247.7146, -43.3736) -> (-245.8075, -45.2808)
  line L256 (-245.5075, -45.2808) -> (-245.2075, -45.2808)
  line L257 (-245.5075, -45.2808) -> (-245.8075, -45.2808)
  line L258 (-248.0075, -42.6665) -> (-248.0075, -25.895)
  line L259 (-243.0075, -25.895) -> (-243.0075, -42.6665)
  arc A102 (-247.7146, -25.1879) -> (-248.0075, -25.895) centre (-247.0075, -25.895) ccw
  line L260 (-247.7146, -25.1879) -> (-245.8075, -23.2808)
  line L261 (-245.5075, -23.2808) -> (-245.8075, -23.2808)
  line L262 (-245.5075, -23.2808) -> (-245.2075, -23.2808)
  arc A103 (-243.0075, -25.895) -> (-243.3004, -25.1879) centre (-244.0075, -25.895) ccw
  line L263 (-243.3004, -25.1879) -> (-245.2075, -23.2808)
  arc A104 (-243.3004, -68.1736) -> (-243.0075, -67.4665) centre (-244.0075, -67.4665) ccw
  arc A105 (-248.0075, -67.4665) -> (-247.7146, -68.1736) centre (-247.0075, -67.4665) ccw
  line L264 (-243.3004, -68.1736) -> (-245.2075, -70.0808)
  line L265 (-247.7146, -68.1736) -> (-245.8075, -70.0808)
  line L266 (-245.5075, -70.0808) -> (-245.2075, -70.0808)
  line L267 (-245.5075, -70.0808) -> (-245.8075, -70.0808)
  line L268 (-248.0075, -67.4665) -> (-248.0075, -50.695)
  line L269 (-243.0075, -50.695) -> (-243.0075, -67.4665)
  arc A106 (-247.7146, -49.9879) -> (-248.0075, -50.695) centre (-247.0075, -50.695) ccw
  line L270 (-247.7146, -49.9879) -> (-245.8075, -48.0808)
  line L271 (-245.5075, -48.0808) -> (-245.8075, -48.0808)
  line L272 (-245.5075, -48.0808) -> (-245.2075, -48.0808)
  arc A107 (-243.0075, -50.695) -> (-243.3004, -49.9879) centre (-244.0075, -50.695) ccw
  line L273 (-243.3004, -49.9879) -> (-245.2075, -48.0808)
  arc A108 (-267.0004, -73.6879) -> (-266.2933, -73.9808) centre (-266.2933, -72.9808) ccw
  arc A109 (-266.2933, -68.9808) -> (-267.0004, -69.2736) centre (-266.2933, -69.9808) ccw
  line L274 (-267.0004, -73.6879) -> (-268.9075, -71.7808)
  line L275 (-267.0004, -69.2736) -> (-268.9075, -71.1808)
  line L276 (-268.9075, -71.4808) -> (-268.9075, -71.7808)
  line L277 (-268.9075, -71.4808) -> (-268.9075, -71.1808)
  line L278 (-266.2933, -68.9808) -> (-249.5217, -68.9808)
  line L279 (-249.5217, -73.9808) -> (-266.2933, -73.9808)
  arc A110 (-248.8146, -69.2736) -> (-249.5217, -68.9808) centre (-249.5217, -69.9808) ccw
  line L280 (-248.8146, -69.2736) -> (-246.9075, -71.1808)
  line L281 (-246.9075, -71.4808) -> (-246.9075, -71.1808)
  line L282 (-246.9075, -71.4808) -> (-246.9075, -71.7808)
  arc A111 (-249.5217, -73.9808) -> (-248.8146, -73.6879) centre (-249.5217, -72.9808) ccw
  line L283 (-248.8146, -73.6879) -> (-246.9075, -71.7808)
  arc A112 (-304.3004, -24.0879) -> (-303.5933, -24.3808) centre (-303.5933, -23.3808) ccw
  arc A113 (-303.5933, -19.3808) -> (-304.3004, -19.6736) centre (-303.5933, -20.3808) ccw
  line L284 (-304.3004, -24.0879) -> (-306.2075, -22.1808)
  line L285 (-304.3004, -19.6736) -> (-306.2075, -21.5808)
  line L286 (-306.2075, -21.8808) -> (-306.2075, -22.1808)
  line L287 (-306.2075, -21.8808) -> (-306.2075, -21.5808)
  line L288 (-303.5933, -19.3808) -> (-286.8217, -19.3808)
  line L289 (-286.8217, -24.3808) -> (-303.5933, -24.3808)
  arc A114 (-286.1146, -19.6736) -> (-286.8217, -19.3808) centre (-286.8217, -20.3808) ccw
  line L290 (-286.1146, -19.6736) -> (-284.2075, -21.5808)
  line L291 (-284.2075, -21.8808) -> (-284.2075, -21.5808)
  line L292 (-284.2075, -21.8808) -> (-284.2075, -22.1808)
  arc A115 (-286.8217, -24.3808) -> (-286.1146, -24.0879) centre (-286.8217, -23.3808) ccw
  line L293 (-286.1146, -24.0879) -> (-284.2075, -22.1808)
  arc A116 (-304.3004, -48.8879) -> (-303.5933, -49.1808) centre (-303.5933, -48.1808) ccw
  arc A117 (-303.5933, -44.1808) -> (-304.3004, -44.4736) centre (-303.5933, -45.1808) ccw
  line L294 (-304.3004, -48.8879) -> (-306.2075, -46.9808)
  line L295 (-304.3004, -44.4736) -> (-306.2075, -46.3808)
  line L296 (-306.2075, -46.6808) -> (-306.2075, -46.9808)
  line L297 (-306.2075, -46.6808) -> (-306.2075, -46.3808)
  line L298 (-303.5933, -44.1808) -> (-286.8217, -44.1808)
  line L299 (-286.8217, -49.1808) -> (-303.5933, -49.1808)
  arc A118 (-286.1146, -44.4736) -> (-286.8217, -44.1808) centre (-286.8217, -45.1808) ccw
  line L300 (-286.1146, -44.4736) -> (-284.2075, -46.3808)
  line L301 (-284.2075, -46.6808) -> (-284.2075, -46.3808)
  line L302 (-284.2075, -46.6808) -> (-284.2075, -46.9808)
  arc A119 (-286.8217, -49.1808) -> (-286.1146, -48.8879) centre (-286.8217, -48.1808) ccw
  line L303 (-286.1146, -48.8879) -> (-284.2075, -46.9808)
  arc A120 (-305.4004, -43.3736) -> (-305.1075, -42.6665) centre (-306.1075, -42.6665) ccw
  arc A121 (-310.1075, -42.6665) -> (-309.8146, -43.3736) centre (-309.1075, -42.6665) ccw
  line L304 (-305.4004, -43.3736) -> (-307.3075, -45.2808)
  line L305 (-309.8146, -43.3736) -> (-307.9075, -45.2808)
  line L306 (-307.6075, -45.2808) -> (-307.3075, -45.2808)
  line L307 (-307.6075, -45.2808) -> (-307.9075, -45.2808)
  line L308 (-310.1075, -42.6665) -> (-310.1075, -25.895)
  line L309 (-305.1075, -25.895) -> (-305.1075, -42.6665)
  arc A122 (-309.8146, -25.1879) -> (-310.1075, -25.895) centre (-309.1075, -25.895) ccw
  line L310 (-309.8146, -25.1879) -> (-307.9075, -23.2808)
  line L311 (-307.6075, -23.2808) -> (-307.9075, -23.2808)
  line L312 (-307.6075, -23.2808) -> (-307.3075, -23.2808)
  arc A123 (-305.1075, -25.895) -> (-305.4004, -25.1879) centre (-306.1075, -25.895) ccw
  line L313 (-305.4004, -25.1879) -> (-307.3075, -23.2808)
  arc A124 (-305.4004, -68.1736) -> (-305.1075, -67.4665) centre (-306.1075, -67.4665) ccw
  arc A125 (-310.1075, -67.4665) -> (-309.8146, -68.1736) centre (-309.1075, -67.4665) ccw
  line L314 (-305.4004, -68.1736) -> (-307.3075, -70.0808)
  line L315 (-309.8146, -68.1736) -> (-307.9075, -70.0808)
  line L316 (-307.6075, -70.0808) -> (-307.3075, -70.0808)
  line L317 (-307.6075, -70.0808) -> (-307.9075, -70.0808)
  line L318 (-310.1075, -67.4665) -> (-310.1075, -50.695)
  line L319 (-305.1075, -50.695) -> (-305.1075, -67.4665)
  arc A126 (-309.8146, -49.9879) -> (-310.1075, -50.695) centre (-309.1075, -50.695) ccw
  line L320 (-309.8146, -49.9879) -> (-307.9075, -48.0808)
  line L321 (-307.6075, -48.0808) -> (-307.9075, -48.0808)
  line L322 (-307.6075, -48.0808) -> (-307.3075, -48.0808)
  arc A127 (-305.1075, -50.695) -> (-305.4004, -49.9879) centre (-306.1075, -50.695) ccw
  line L323 (-305.4004, -49.9879) -> (-307.3075, -48.0808)
  arc A128 (-280.6004, -43.3736) -> (-280.3075, -42.6665) centre (-281.3075, -42.6665) ccw
  arc A129 (-285.3075, -42.6665) -> (-285.0146, -43.3736) centre (-284.3075, -42.6665) ccw
  line L324 (-280.6004, -43.3736) -> (-282.5075, -45.2808)
  line L325 (-285.0146, -43.3736) -> (-283.1075, -45.2808)
  line L326 (-282.8075, -45.2808) -> (-282.5075, -45.2808)
  line L327 (-282.8075, -45.2808) -> (-283.1075, -45.2808)
  line L328 (-285.3075, -42.6665) -> (-285.3075, -25.895)
  line L329 (-280.3075, -25.895) -> (-280.3075, -42.6665)
  arc A130 (-285.0146, -25.1879) -> (-285.3075, -25.895) centre (-284.3075, -25.895) ccw
  line L330 (-285.0146, -25.1879) -> (-283.1075, -23.2808)
  line L331 (-282.8075, -23.2808) -> (-283.1075, -23.2808)
  line L332 (-282.8075, -23.2808) -> (-282.5075, -23.2808)
  arc A131 (-280.3075, -25.895) -> (-280.6004, -25.1879) centre (-281.3075, -25.895) ccw
  line L333 (-280.6004, -25.1879) -> (-282.5075, -23.2808)
  arc A132 (-280.6004, -68.1736) -> (-280.3075, -67.4665) centre (-281.3075, -67.4665) ccw
  arc A133 (-285.3075, -67.4665) -> (-285.0146, -68.1736) centre (-284.3075, -67.4665) ccw
  line L334 (-280.6004, -68.1736) -> (-282.5075, -70.0808)
  line L335 (-285.0146, -68.1736) -> (-283.1075, -70.0808)
  line L336 (-282.8075, -70.0808) -> (-282.5075, -70.0808)
  line L337 (-282.8075, -70.0808) -> (-283.1075, -70.0808)
  line L338 (-285.3075, -67.4665) -> (-285.3075, -50.695)
  line L339 (-280.3075, -50.695) -> (-280.3075, -67.4665)
  arc A134 (-285.0146, -49.9879) -> (-285.3075, -50.695) centre (-284.3075, -50.695) ccw
  line L340 (-285.0146, -49.9879) -> (-283.1075, -48.0808)
  line L341 (-282.8075, -48.0808) -> (-283.1075, -48.0808)
  line L342 (-282.8075, -48.0808) -> (-282.5075, -48.0808)
  arc A135 (-280.3075, -50.695) -> (-280.6004, -49.9879) centre (-281.3075, -50.695) ccw